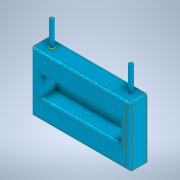
# Autodesk Inventor part: part3nn
Saved by Autodesk Inventor 2021.3 (Build 253353000, 353)
## iProperties
Created: 2021-07-06
Part Number: part3nn
Material: Polyethylene, High Density
Document SubType Name: Modeling
Designer: ASUS
Density: 0.952 g/cm^3
Appearance: Smooth - Off-White
Author: ASUS
Autodesk Inventor part; units mm, degrees
ref_plane "YZ Plane" through (0, 0, 0) normal (1, 0, 0) x (0, 1, 0)
ref_plane "XZ Plane" through (0, 0, 0) normal (0, 1, 0) x (-1, 0, 0)
ref_plane "XY Plane" through (0, 0, 0) normal (0, 0, 1) x (1, 0, 0)
sketch "Sketch1" plane through (0, 0, 0) normal (0, 0, 1) x (1, 0, 0)
  line L0 (0, 60) -> (0, 0)
  line L1 (0, 0) -> (100, 0)
  line L2 (100, 0) -> (100, 60)
  line L3 (100, 60) -> (0, 60)
  constraints: 8 end point, 3 perpendicular, 1 vertical
extrude "Extrusion1" add sketch "Sketch1" along normal blind 20
sketch "Sketch2" plane through (0, 0, 20) normal (0, 0, 1) x (1, 0, 0)
  line L0 (10, 40) -> (90, 40)
  line L1 (90, 40) -> (90, 20)
  line L2 (90, 20) -> (10, 20)
  line L3 (10, 20) -> (10, 40)
  line L4 (100, 60) -> (0, 60) projected
  line L5 (0, 0) -> (100, 0) projected
  line L6 (100, 0) -> (100, 60) projected
  line L7 (0, 60) -> (0, 0) projected
  constraints: 8 end point, 2 parallel, 1 horizontal, 1 perpendicular
extrude "Extrusion2" cut sketch "Sketch2" against normal blind 15 contours L0 L1 L2 L3
sketch "Sketch3" plane through (0, 0, 20) normal (0, 0, 1) x (1, 0, 0)
  line L0 (38.6013, 31.0426) -> (51.4646, 31.0426)
  line L1 (51.4646, 31.0426) -> (51.4646, 28.004)
  line L2 (51.4646, 28.004) -> (38.6013, 28.004)
  line L3 (38.6013, 28.004) -> (38.6013, 31.0426)
  point P0 (0, 0)
  constraints: 8 end point, 2 parallel, 1 horizontal, 1 perpendicular
extrude "Extrusion3" cut sketch "Sketch3" against normal through all
sketch "Sketch4" plane through (0, 60, 0) normal (0, 1, 0) x (1, 0, 0)
  line L0 (0, 0) -> (0, -20) projected
  line L1 (100, 0) -> (100, -20) projected
  circle A0 centre (10.2828, -8.9975) radius 2.1128
  circle A1 centre (90.2822, -8.6847) radius 2.1128
  dimension "d18" = 80
  constraints: 2 centre point
  measures "d18" distance of A1.centre A0.centre
extrude "Extrusion4" add sketch "Sketch4" along normal blind 25
sketch "Sketch5" plane through (0, 60, 0) normal (0, 1, 0) x (1, 0, 0)
  circle A0 centre (10.2828, -8.9975) radius 2.1128 projected
  line L0 (97.4061, -6.1607) -> (97.5, -6.1584)
  line L1 (10.2828, -5.156) -> (10.2828, -8.9975)
  point P0 (0, 0)
  constraints: 4 end point
fillet "Fillet1" radius 3 13 edges at (50, 60, 20) (100, 30, 20) (100, 60, 10) (100, 30, 0) (50, 60, 0) (50, 0, 20) (50, 20, 20) (50, 40, 20) (10, 30, 20) (90, 30, 20) (0, 30, 20) (0, 30, 0) (50, 0, 0)
body "Solid1"
